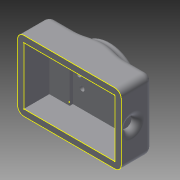
# Autodesk Inventor part: ładowarka usb v2
Saved by Autodesk Inventor 2014 (Build 180170000, 170)
## iProperties
Created: 2017-04-11
Part Number: ładowarka usb v2
Material: Ogólny
Document SubType Name: Modeling
Designer: hpdc7700
Density: 1 g/cm^3
Appearance: Domyślna
Author: hpdc7700
Autodesk Inventor part; units mm, degrees
ref_plane "YZ Plane" through (0, 0, 0) normal (1, 0, 0) x (0, 1, 0)
ref_plane "XZ Plane" through (0, 0, 0) normal (0, 1, 0) x (-1, 0, 0)
ref_plane "XY Plane" through (0, 0, 0) normal (0, 0, 1) x (1, 0, 0)
sketch "Szkic1" plane through (0, 0, 0) normal (0, 1, 0) x (-1, 0, 0)
  circle A0 centre (0, 0) radius 10
  circle A1 centre (0, 0) radius 10
  dimension "d0" = 20
  dimension "d1" = 20
  constraints: 2 centre point, 2 coincident
  measures "d0" diameter of A0
  measures "d1" diameter of A1
extrude "Wyciągnięcie proste1" add sketch "Szkic1" along normal blind 3
sketch "Szkic2" plane through (0, 3, 0) normal (0, 1, 0) x (1, 0, 0)
  circle A0 centre (-6, -0.0067) radius 0.75
  circle A1 centre (-4.9753, -3.3535) radius 0.75
  circle A2 centre (-4.983, 3.3423) radius 0.75
  line L0 (0.0051, -9.2479) -> (-0.004, 7.2751)
  point P0 (0, 0)
  dimension "d4" = 1.5
  dimension "d5" = 1.5
  dimension "d6" = 1.5
  dimension "d7" = 1.017
  dimension "d8" = 1.0247
  dimension "d9" = 4.9772
  dimension "d10" = 6
  dimension "d11" = 4.9812
  dimension "d44" = 3.349
  dimension "d45" = 3.3468
  constraints: 3 centre point, 2 end point
  measures "d4" diameter of A0
  measures "d5" diameter of A1
  measures "d6" diameter of A2
  measures "d7" horizontal distance of A2.centre A0.centre
  measures "d8" horizontal distance of A0.centre A1.centre
  measures "d9" distance from line of L0 A1.centre
  measures "d10" distance from line of L0 A0.centre
  measures "d11" distance from line of L0 A2.centre
  measures "d44" vertical distance of A0.centre A2.centre
  measures "d45" vertical distance of A0.centre A1.centre
extrude "Wyciągnięcie proste2" cut sketch "Szkic2" against normal up to surface (3 mm away)
sketch "Szkic3" plane through (0, 3, 0) normal (0, 1, 0) x (1, 0, 0)
  circle A0 centre (0, -6) radius 2.5
  circle A1 centre (0, 6) radius 2.5
  circle A2 centre (0, 0) radius 10
  dimension "d14" = 5
  dimension "d15" = 5
  dimension "d46" = 6
  dimension "d47" = 6
  constraints: 3 centre point
  measures "d14" diameter of A1
  measures "d15" diameter of A0
  measures "d46" distance of A2.centre A1.centre
  measures "d47" distance of A2.centre A0.centre
extrude "Wyciągnięcie proste3" cut sketch "Szkic3" against normal blind 2.5 contours A0 | A1
chamfer "Faza1" distance 0.4 angle 45 2 edges at (-2.5, 3, -6) (-2.5, 3, 6)
chamfer "Faza2" distance 0.4 angle 45 3 edges at (-5.7253, 3, 3.3535) (-6.75, 3, 0.0067) (-5.733, 3, -3.3423)
sketch "Szkic4" plane through (0, 0, 0) normal (0, -1, 0) x (1, 0, 0)
  circle A0 centre (-4.9753, 3.3535) radius 0.75 projected
  circle A1 centre (-4.983, -3.3423) radius 0.75 projected
  circle A2 centre (-6, 0.0067) radius 0.75 projected
  circle A3 centre (0, 0) radius 10 projected
  line L0 (14.25, -9) -> (14.25, 9)
  line L1 (-14.25, 9) -> (-14.25, -9)
  line L2 (-14.25, -9) -> (14.25, 9) construction
  line L3 (14.25, -9) -> (-14.25, 9) construction
  line L4 (-16.25, -11) -> (16.25, -11)
  line L5 (16.25, -11) -> (16.25, 11)
  line L6 (16.25, 11) -> (-16.25, 11)
  line L7 (-16.25, 11) -> (-16.25, -11)
  line L8 (-16.25, -11) -> (16.25, 11) construction
  line L9 (16.25, -11) -> (-16.25, 11) construction
  circle A4 centre (-4.9753, 3.3535) radius 0.75
  circle A5 centre (-6, 0.0067) radius 0.75
  circle A6 centre (-4.983, -3.3423) radius 0.75
  circle A7 centre (-4.9753, 3.3535) radius 0.75 projected
  circle A8 centre (-4.983, -3.3423) radius 0.75 projected
  circle A9 centre (-6, 0.0067) radius 0.75 projected
  circle A10 centre (0, 0) radius 10 projected
  line L10 (14.25, 9) -> (4.3589, 9)
  line L11 (-4.3589, 9) -> (-14.25, 9)
  line L12 (-14.25, -9) -> (-4.3589, -9)
  line L13 (4.3589, -9) -> (14.25, -9)
  dimension "d24" = 28.5
  dimension "d25" = 18
  dimension "d26" = 2
  constraints: 28 end point, 7 parallel, 4 midpoint, 4 point on circle, 3 centre point, 3 coincident, 3 concentric, 3 horizontal, 3 perpendicular
  measures "d24" distance of L1.start L0.end
  measures "d25" distance of L0.end L0.start
  measures "d26" distance between parallel lines of L7 L1
extrude "Wyciągnięcie proste4" add sketch "Szkic4" along normal blind 2 contours A3 | A3 L10 L0 L13 | A3 L12 L1 L11 | L7 L6 L5 L4
sketch "Szkic5" plane through (0, -2, 0) normal (0, -1, 0) x (1, 0, 0)
  line L0 (-16.25, -11) -> (16.25, -11) projected
  line L1 (16.25, -11) -> (16.25, 11) projected
  line L2 (16.25, 11) -> (-16.25, 11) projected
  line L3 (-16.25, 11) -> (-16.25, -11) projected
  line L4 (-14.2536, -9) -> (14.2464, -9)
  line L5 (14.2464, -9) -> (14.2464, 9)
  line L6 (14.2464, 9) -> (-14.2536, 9)
  line L7 (-14.2536, 9) -> (-14.2536, -9)
  line L8 (-14.2536, -9) -> (14.2464, 9) construction
  line L9 (14.2464, -9) -> (-14.2536, 9) construction
  circle A0 centre (-6, 0.0067) radius 0.75 projected
  circle A1 centre (-4.983, -3.3423) radius 0.75 projected
  circle A2 centre (-4.9753, 3.3535) radius 0.75 projected
  line L10 (-16.25, -11) -> (16.25, -11) projected
  line L11 (16.25, -11) -> (16.25, 11) projected
  line L12 (16.25, 11) -> (-16.25, 11) projected
  line L13 (-16.25, 11) -> (-16.25, -11) projected
  point P0 (0, 0)
  point P1 (-0.0036, 0)
  dimension "d30" = 28.5
  dimension "d31" = 18
  constraints: 12 end point, 2 midpoint, 2 parallel, 1 horizontal, 1 perpendicular
  measures "d30" distance of L6.end L5.end
  measures "d31" distance of L5.end L4.end
extrude "Wyciągnięcie proste5" add sketch "Szkic5" along normal blind 8 contours L3 L2 L1 L0
fillet "Zaokrąglenie1" radius 2 5 edges at (10, 0, 0) (0, 0, -11) (16.25, 0, 0) (0, 0, 11) (-16.25, 0, 0)
fillet "Zaokrąglenie2" radius 1 1 edges at (10, 3, 0)
fillet "Zaokrąglenie3" radius 2 8 edges at (-15.6642, -0.5858, 10.4142) (-16.25, -6, 11) (-15.6642, -0.5858, -10.4142) (-16.25, -6, -11) (15.6642, -0.5858, 10.4142) (16.25, -6, 11) (15.6642, -0.5858, -10.4142) (16.25, -6, -11)
sketch "Szkic6" plane through (0, -2, 0) normal (0, -1, 0) x (1, 0, 0)
  line L0 (-14.2536, -9) -> (14.2464, -9) projected
  circle A0 centre (-6, 0.0067) radius 0.75 projected
  circle A1 centre (-4.983, -3.3423) radius 0.75 projected
  circle A2 centre (-4.9753, 3.3535) radius 0.75 projected
  line L1 (-7.872, 9) -> (7.872, 9)
  line L2 (7.872, 9) -> (7.872, -9)
  line L3 (7.872, -9) -> (-7.872, -9)
  line L4 (-7.872, -9) -> (-7.872, 9)
  line L5 (-7.872, 9) -> (7.872, -9) construction
  line L6 (7.872, 9) -> (-7.872, -9) construction
  point P0 (0, 0)
  constraints: 12 end point, 2 midpoint, 2 parallel, 1 horizontal, 1 perpendicular, 1 point on line
extrude "Wyciągnięcie proste6" cut sketch "Szkic6" against normal blind 1
sketch "Szkic7" plane through (16.25, -10, -9) normal (1, 0, 0) x (0, 0, -1)
  circle A0 centre (-9, 3.5) radius 1.75
  point P0 (-9, 10)
  dimension "d39" = 3.5
  dimension "d43" = 6.5
  constraints: 1 centre point
  measures "d39" diameter of A0
  measures "d43" distance of point (-9, 10) A0.centre
extrude "Wyciągnięcie proste7" cut sketch "Szkic7" against normal blind 2
fillet "Zaokrąglenie4" radius 2 1 edges at (16.25, -6.5, 1.75)
sketch "Szkic8" plane through (0, -10, 0) normal (0, -1, 0) x (1, 0, 0)
  line L0 (16.25, 1.3463) -> (16.25, 9) projected
  arc A0 (16.25, 9) -> (14.25, 11) centre (14.25, 9) ccw projected
  line L1 (14.25, 11) -> (-14.25, 11) projected
  arc A1 (-14.25, 11) -> (-16.25, 9) centre (-14.25, 9) ccw projected
  line L2 (-16.25, 9) -> (-16.25, -9) projected
  arc A2 (-16.25, -9) -> (-14.25, -11) centre (-14.25, -9) ccw projected
  line L3 (-14.25, -11) -> (14.25, -11) projected
  arc A3 (14.25, -11) -> (16.25, -9) centre (14.25, -9) ccw projected
  line L4 (16.25, -9) -> (16.25, -1.3463) projected
  line L5 (-14.2536, -9) -> (-14.2536, 9) projected
  line L6 (-14.2536, 9) -> (14.2464, 9) projected
  line L7 (14.2464, 9) -> (14.2464, -9) projected
  line L8 (14.2464, -9) -> (-14.2536, -9) projected
  line L9 (16.25, 1.3463) -> (16.25, 9) projected
  arc A4 (16.25, 9) -> (14.25, 11) centre (14.25, 9) ccw projected
  line L10 (14.25, 11) -> (-14.25, 11) projected
  arc A5 (-14.25, 11) -> (-16.25, 9) centre (-14.25, 9) ccw projected
  line L11 (-16.25, 9) -> (-16.25, -9) projected
  arc A6 (-16.25, -9) -> (-14.25, -11) centre (-14.25, -9) ccw projected
  line L12 (-14.25, -11) -> (14.25, -11) projected
  arc A7 (14.25, -11) -> (16.25, -9) centre (14.25, -9) ccw projected
  line L13 (16.25, -9) -> (16.25, -1.3463) projected
  line L14 (-14.2536, -9) -> (-14.2536, 9) projected
  line L15 (-14.2536, 9) -> (14.2464, 9) projected
  line L16 (14.2464, 9) -> (14.2464, -9) projected
  line L17 (14.2464, -9) -> (-14.2536, -9) projected
  point P0 (0, 0)
  constraints: 2 vertical alignment
